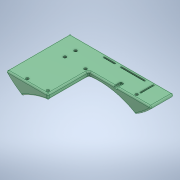
# Autodesk Inventor part: mainboard_mount
Saved by Autodesk Inventor 2020.2 (Build 242310000, 310)
## iProperties
Created: 2020-04-10
Part Number: mainboard_mount
Material: Wood (Birch)
Document SubType Name: Modeling
Designer: agmlego
Mass: 51.9794 g
Surface Area: 215.115 cm^2
Volume: 94.5079 cm^3
Density: 0.55 g/cm^3
Appearance: Smooth - Dark Sea Green
Author: agmlego
Autodesk Inventor part; units mm, degrees
ref_plane "YZ Plane" through (0, 0, 0) normal (1, 0, 0) x (0, 1, 0)
ref_plane "XZ Plane" through (0, 0, 0) normal (0, 1, 0) x (-1, 0, 0)
ref_plane "XY Plane" through (0, 0, 0) normal (0, 0, 1) x (1, 0, 0)
sketch "Sketch1" plane through (0, 0, 0) normal (0, 0, 1) x (1, 0, 0)
  line L0 (-75.8612, 0) -> (75.8612, 0)
  arc A0 (51.3869, -20.32) -> (-51.3869, -20.32) centre (0, -107.1118) ccw
  line L1 (0, 0) -> (0, -107.1118) construction
  arc A1 (-75.8612, 0) -> (-51.3869, -20.32) centre (0, 66.4718) ccw
  arc A2 (51.3869, -20.32) -> (75.8612, 0) centre (0, 66.4718) ccw
  dimension "d1" = 66.4718
  dimension "d2" = 100.8634
  dimension "d3" = 20.32
  constraints: 6 point on circle, 5 end point, 3 centre point, 2 equal radius, 1 horizontal, 1 midpoint, 1 vertical
  measures "d1" distance from line of L0 A1.centre
  measures "d2" radius of A0
  measures "d3" distance from line of L0 A0.end
extrude "Base" add sketch "Sketch1" along normal blind 90
sketch "Sketch2" plane through (-75.8612, 0, 0) normal (0, 1, 0) x (1, 0, 0)
  line L0 (127.8612, -90) -> (23.8612, -90) construction
  line L1 (23.8612, -90) -> (23.8612, 0) construction
  line L2 (23.8612, 0) -> (127.8612, 0) construction
  line L3 (127.8612, 0) -> (127.8612, -90) construction
  line L4 (75.8612, 0) -> (75.8612, -90) construction
  line L5 (151.7224, -90) -> (0, -90) projected
  line L6 (60.8412, -89.37) -> (23.8412, -89.37) construction
  line L7 (23.8412, -89.37) -> (23.8412, -28.37) construction
  line L8 (23.8412, -28.37) -> (60.8412, -28.37) construction
  line L9 (60.8412, -28.37) -> (60.8412, -89.37) construction
  circle A0 centre (27.8412, -85.37) radius 4 construction
  circle A1 centre (27.8412, -32.37) radius 4 construction
  circle A2 centre (56.8412, -85.37) radius 4 construction
  circle A3 centre (56.8412, -32.37) radius 4 construction
  point P0 (27.7852, -17.3228)
  point P1 (124.3052, -27.559)
  dimension "d6" = 90
  dimension "d7" = 104
  dimension "d8" = 3.556
  dimension "d9" = 27.559
  dimension "d10" = 17.3228
  dimension "d11" = 100.076
  dimension "d14" = 61
  dimension "d15" = 37
  dimension "d16" = 8
  dimension "d17" = 104.02
  dimension "d18" = 28.37
  constraints: 18 end point, 8 tangent, 4 centre point, 4 coincident, 4 midpoint, 4 parallel, 3 equal radius, 2 horizontal, 2 perpendicular, 1 point on line
  measures "d6" distance of L0.end L1.end
  measures "d7" distance of L0.start L0.end
  measures "d8" distance from line of L3 point (124.305, -27.559)
  measures "d9" distance from line of L2 point (124.305, -27.559)
  measures "d10" distance from line of L2 point (27.785, -17.323)
  measures "d11" distance from line of L3 point (27.785, -17.323)
  measures "d14" distance of L8.end L6.start
  measures "d15" distance of L7.end L8.end
  measures "d16" diameter of A0
  measures "d17" distance between parallel lines of L3 L7
  measures "d18" distance between parallel lines of L2 L8
hole "Mounting" at (-48.076, 0, 17.3228) at (48.444, 0, 27.559) at (-48.02, 0, 85.37) at (-48.02, 0, 32.37) at (-19.02, 0, 32.37) at (-19.02, 0, 85.37) direction (0, -1, 0) diameter 4.0386 depth 5.7 start extended yes
sketch "Sketch3" plane through (-75.8612, 0, 0) normal (0, 1, 0) x (1, 0, 0)
  line L0 (151.7224, 0) -> (151.7224, -90) projected
  line L1 (151.7224, -90) -> (61.5524, -90)
  line L2 (61.5524, -90) -> (61.5524, -32.7738)
  line L3 (61.5524, -32.7738) -> (151.7224, -32.7738)
  line L4 (151.7224, -32.7738) -> (151.7224, -90)
  point P0 (75.8612, 0)
  dimension "d26" = 90.17
  dimension "d27" = 57.2262
  constraints: 8 end point, 2 parallel, 1 horizontal, 1 perpendicular
  measures "d26" distance of L2.end L3.end
  measures "d27" distance of L1.end L2.end
extrude "G2 Knockout" cut sketch "Sketch3" against normal through all
sketch "Sketch4" plane through (-75.8612, 0, 0) normal (0, 1, 0) x (1, 0, 0)
  line L0 (125.771, -23.3298) -> (123.8914, -23.3298)
  line L1 (123.8914, -23.3298) -> (123.8914, -3.6702)
  line L2 (123.8914, -3.6702) -> (125.771, -3.6702)
  line L3 (125.771, -3.6702) -> (125.771, -23.3298)
  line L4 (113.891, -6.1498) -> (79.0614, -6.1498)
  line L5 (79.0614, -6.1498) -> (79.0614, -4.2702)
  line L6 (79.0614, -4.2702) -> (113.891, -4.2702)
  line L7 (113.891, -4.2702) -> (113.891, -6.1498)
  line L8 (71.801, -6.1498) -> (54.9514, -6.1498)
  line L9 (54.9514, -6.1498) -> (54.9514, -4.2702)
  line L10 (54.9514, -4.2702) -> (71.801, -4.2702)
  line L11 (71.801, -4.2702) -> (71.801, -6.1498)
  line L12 (102.271, -32.7898) -> (97.5414, -32.7898)
  line L13 (97.5414, -32.7898) -> (97.5414, -23.2902)
  line L14 (97.5414, -23.2902) -> (102.271, -23.2902)
  line L15 (102.271, -23.2902) -> (102.271, -32.7898)
  circle A0 centre (124.8312, -22.39) radius 0.9398 construction
  circle A1 centre (124.8312, -4.61) radius 0.9398 construction
  circle A2 centre (101.3312, -31.85) radius 0.9398 construction
  circle A3 centre (98.4812, -31.85) radius 0.9398 construction
  circle A4 centre (98.4812, -24.23) radius 0.9398 construction
  circle A5 centre (101.3312, -24.23) radius 0.9398 construction
  circle A6 centre (112.9512, -5.21) radius 0.9398 construction
  circle A7 centre (80.0012, -5.21) radius 0.9398 construction
  circle A8 centre (70.8612, -5.21) radius 0.9398 construction
  circle A9 centre (55.8912, -5.21) radius 0.9398 construction
  circle A10 centre (124.3052, -27.559) radius 2.0193 construction
  circle A11 centre (110.9512, -5.21) radius 0.9398 construction
  line L16 (112.9512, -5.21) -> (110.9512, -5.21) construction
  line L17 (111.9512, -6.1498) -> (111.9512, -4.2702) construction
  circle A12 centre (82.0012, -5.21) radius 0.9398 construction
  line L18 (82.0012, -5.21) -> (80.0012, -5.21) construction
  line L19 (81.0012, -6.1498) -> (81.0012, -4.2702) construction
  circle A13 centre (68.8612, -5.21) radius 0.9398 construction
  circle A14 centre (57.8912, -5.21) radius 0.9398 construction
  line L20 (57.8912, -5.21) -> (55.8912, -5.21) construction
  line L21 (70.8612, -5.21) -> (68.8612, -5.21) construction
  line L22 (69.8612, -6.1498) -> (69.8612, -4.2702) construction
  line L23 (56.8912, -6.1498) -> (56.8912, -4.2702) construction
  point P0 (75.8612, 0)
  point P1 (127.8612, 0)
  point P2 (111.9512, -5.21)
  point P3 (81.0012, -5.21)
  point P4 (69.8612, -5.21)
  point P5 (56.8912, -5.21)
  dimension "d30" = 1.8796
  dimension "d32" = 27.559
  dimension "d33" = 3.556
  dimension "d34" = 22.39
  dimension "d35" = 3.03
  dimension "d36" = 26.53
  dimension "d37" = 31.85
  dimension "d38" = 29.38
  dimension "d39" = 5.21
  dimension "d40" = 2
  dimension "d41" = 15.91
  dimension "d42" = 46.86
  dimension "d43" = 58
  dimension "d44" = 70.97
  dimension "d45" = 7.62
  dimension "d46" = 17.78
  constraints: 48 end point, 26 tangent, 14 centre point, 12 equal radius, 10 point on line, 9 parallel, 8 midpoint, 7 horizontal, 6 perpendicular, 3 collinear, 1 vertical
  measures "d30" diameter of A0
  measures "d32" vertical distance of point (127.861, 0) A10.centre
  measures "d33" horizontal distance of point (127.861, 0) A10.centre
  measures "d34" vertical distance of point (127.861, 0) A0.centre
  measures "d35" horizontal distance of point (127.861, 0) A0.centre
  measures "d36" horizontal distance of point (127.861, 0) A2.centre
  measures "d37" vertical distance of point (127.861, 0) A2.centre
  measures "d38" horizontal distance of point (127.861, 0) A3.centre
  measures "d39" vertical distance of point (127.861, 0) L16.start
  measures "d40" distance of L16.start L16.end
  measures "d41" distance from line of point (127.861, 0) L17
  measures "d42" distance from line of point (127.861, 0) L19
  measures "d43" distance from line of point (127.861, 0) L22
  measures "d44" distance from line of point (127.861, 0) L23
  measures "d45" distance of A4.centre A3.centre
  measures "d46" distance of A1.centre A0.centre
extrude "Pin Clearance" cut sketch "Sketch4" against normal blind 2.54
fillet "Fillet1" radius 0.9398 29 edges at (-12.485, -2.54, 4.2702) (-12.485, -2.54, 6.1498) (-20.9098, -2.54, 5.21) (-20.9098, -1.27, 6.1498) (-20.9098, -1.27, 4.2702) (-4.0602, -2.54, 5.21) (-4.0602, -1.27, 4.2702) (-4.0602, -1.27, 6.1498) (3.2002, -1.27, 6.1498) (3.2002, -1.27, 4.2702) (3.2002, -2.54, 5.21) (20.615, -2.54, 4.2702) (20.615, -2.54, 6.1498) (38.0298, -1.27, 4.2702) (38.0298, -2.54, 5.21) (38.0298, -1.27, 6.1498) (48.0302, -1.27, 3.6702) (48.97, -2.54, 3.6702) (49.9098, -1.27, 3.6702) (49.9098, -2.54, 13.5) (48.0302, -2.54, 13.5) (48.0302, -1.27, 23.3298) (48.97, -2.54, 23.3298) (49.9098, -1.27, 23.3298) (21.6802, -1.27, 23.2902) (26.4098, -1.27, 23.2902) (24.045, -2.54, 23.2902) (21.6802, -2.54, 28.032) (26.4098, -2.54, 28.032)
fillet "Fillet2" radius 2 19 edges at (-33.4898, -11.9705, 90) (-14.3088, -3.6343, 90) (-14.3088, -7.2685, 61.3869) (-14.3088, -3.6343, 32.7738) (19.654, -8.1818, 32.7738) (0, -6.2484, 0) (-51.3869, -20.32, 45) (51.3869, -20.32, 16.3869) (-75.8612, 0, 45) (75.8612, 0, 16.3869) (64.4301, -11.1309, 32.7738) (51.1355, 0, 32.7738) (-64.4301, -11.1309, 90) (-45.085, 0, 90) (-14.3088, 0, 61.3869) (3.6857, 0, 32.7738) (0, 0, 0) (-64.4301, -11.1309, 0) (64.4301, -11.1309, 0)
equation "\"d2\" = 0.5 * hull_id"
equation "\"hull_od\" = 219.075"
equation "\"hull_id\" = 201.7268"
equation "\"hull_wall\" = 8.6741"
equation "\"hull_length\" = 609.6"
equation "\"hull_spacing\" = 390.525"
equation "\"impeller_od\" = 76.2"
equation "\"impeller_clearance\" = 0.5"
equation "\"impeller_shaft_id\" = 3.175"
equation "\"impeller_shaft_od\" = 5.715"
equation "\"impeller_shaft_support\" = 3.175"
equation "\"impeller_intake_od\" = 19.05"
equation "\"impeller_vane_thick\" = 2"
equation "\"impeller_vane_inner_rad\" = 3.175"
equation "\"impeller_vane_outer_rad\" = 0.37206"
equation "\"magnet_od\" = 5.95"
equation "\"magnet_clearance\" = 0.25"
equation "\"magnet_rad\" = 0.25"
equation "\"magnet_circle_offset\" = 3.175"
equation "\"motor_shaft_od\" = 12.7"
equation "\"motor_shaft_length\" = 31.75"
equation "\"motor_shaft_key\" = 3.048"
equation "\"d0\" = hull_id"
body "Solid1"
